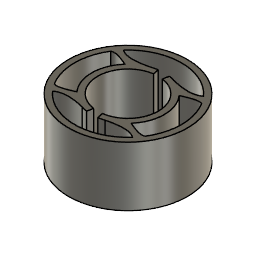
HeadTest (Autodesk Fusion 360 archive; units mm, degrees)
design "ReverseCoupler"
Autodesk Fusion 360 part; units mm, degrees
sketch "Sketch1" plane through (0, 0, 0) normal (0, 0, 1) x (1, 0, 0)
  circle A0 centre (0, 0) radius 5
  circle A1 centre (0, 0) radius 4.5
  line L0 (-6, 0) -> (8, 0) construction
  line L1 (0, -6.5) -> (0, 7.6827) construction
  line L2 (-0.3675, 2.5234) -> (-0.474, 3.0129)
  line L3 (-0.3675, -2.5234) -> (-0.474, -3.0129)
  line L4 (0.3675, -2.5234) -> (0.474, -3.0129)
  line L5 (0.3675, 2.5234) -> (0.474, 3.0129)
  arc A2 (-0.3675, 2.5234) -> (-0.3675, -2.5234) centre (0, 0) ccw
  arc A3 (0.3675, -2.5234) -> (0.3675, 2.5234) centre (0, 0) ccw
  arc A4 (-0.474, 3.0129) -> (-0.474, -3.0129) centre (0, 0) ccw
  arc A5 (0.474, -3.0129) -> (0.474, 3.0129) centre (0, 0) ccw
  spline S0 degree 5 poles (-0.9612, 2.8946) (-1.0282, 2.8783) (-1.1605, 2.8471) (-1.3543, 2.8051) (-1.6029, 2.7584) (-1.8962, 2.7168) (-2.1703, 2.6936) (-2.4235, 2.6906) (-2.6543, 2.7092) (-2.8628, 2.7492) (-3.0505, 2.8093) (-3.1851, 2.8722) (-3.2779, 2.9273) (-3.3362, 2.9674) (-3.3645, 2.9883) knots 0 0 0 0 0 0 0.1 0.2 0.3 0.4 0.5 0.6 0.7 0.8 0.9 1 1 1 1 1 1
  spline S1 degree 5 poles (-2.2886, 2.0162) (-2.3369, 2.0378) (-2.4322, 2.0797) (-2.5706, 2.1389) (-2.7462, 2.2105) (-2.9496, 2.2866) (-3.1354, 2.3481) (-3.3018, 2.3935) (-3.4472, 2.4215) (-3.5716, 2.4322) (-3.6763, 2.4265) (-3.7453, 2.4097) (-3.7893, 2.3907) (-3.8152, 2.3752) (-3.8273, 2.3668) knots 0 0 0 0 0 0 0.1 0.2 0.3 0.4 0.5 0.6 0.7 0.8 0.9 1 1 1 1 1 1
  spline S2 degree 5 poles (-0.9612, -2.8946) (-1.0282, -2.8783) (-1.1605, -2.8471) (-1.3543, -2.8051) (-1.6029, -2.7584) (-1.8962, -2.7168) (-2.1703, -2.6936) (-2.4235, -2.6906) (-2.6543, -2.7092) (-2.8628, -2.7492) (-3.0505, -2.8093) (-3.1851, -2.8722) (-3.2779, -2.9273) (-3.3362, -2.9674) (-3.3645, -2.9883) knots 0 0 0 0 0 0 0.1 0.2 0.3 0.4 0.5 0.6 0.7 0.8 0.9 1 1 1 1 1 1
  line L6 (-0.6756, 2.9642) -> (-1.2467, 2.825)
  line L7 (-3.1897, 2.8588) -> (-3.5393, 3.1178)
  line L8 (-0.6756, -2.9642) -> (-1.2467, -2.825)
  line L9 (-3.1897, -2.8588) -> (-3.5393, -3.1178)
  spline S3 degree 5 poles (-2.2886, -2.0162) (-2.3369, -2.0378) (-2.4322, -2.0797) (-2.5706, -2.1389) (-2.7462, -2.2105) (-2.9496, -2.2866) (-3.1354, -2.3481) (-3.3018, -2.3935) (-3.4472, -2.4215) (-3.5716, -2.4322) (-3.6763, -2.4265) (-3.7453, -2.4097) (-3.7893, -2.3907) (-3.8152, -2.3752) (-3.8273, -2.3668) knots 0 0 0 0 0 0 0.1 0.2 0.3 0.4 0.5 0.6 0.7 0.8 0.9 1 1 1 1 1 1
  line L10 (-2.0941, 1.9294) -> (-2.483, 2.1029)
  line L11 (-3.7334, 2.4323) -> (-3.9212, 2.3013)
  line L12 (-2.0941, -1.9294) -> (-2.483, -2.1029)
  line L13 (-3.7334, -2.4323) -> (-3.9212, -2.3013)
  spline S4 degree 5 poles (0.9612, 2.8946) (1.0282, 2.8783) (1.1605, 2.8471) (1.3543, 2.8051) (1.6029, 2.7584) (1.8962, 2.7168) (2.1703, 2.6936) (2.4235, 2.6906) (2.6543, 2.7092) (2.8628, 2.7492) (3.0505, 2.8093) (3.1851, 2.8722) (3.2779, 2.9273) (3.3362, 2.9674) (3.3645, 2.9883) knots 0 0 0 0 0 0 0.1 0.2 0.3 0.4 0.5 0.6 0.7 0.8 0.9 1 1 1 1 1 1
  line L14 (0.6756, 2.9642) -> (1.2467, 2.825)
  line L15 (3.1897, 2.8588) -> (3.5393, 3.1178)
  spline S5 degree 5 poles (2.2886, 2.0162) (2.3369, 2.0378) (2.4322, 2.0797) (2.5706, 2.1389) (2.7462, 2.2105) (2.9496, 2.2866) (3.1354, 2.3481) (3.3018, 2.3935) (3.4472, 2.4215) (3.5716, 2.4322) (3.6763, 2.4265) (3.7453, 2.4097) (3.7893, 2.3907) (3.8152, 2.3752) (3.8273, 2.3668) knots 0 0 0 0 0 0 0.1 0.2 0.3 0.4 0.5 0.6 0.7 0.8 0.9 1 1 1 1 1 1
  line L16 (2.0941, 1.9294) -> (2.483, 2.1029)
  line L17 (3.7334, 2.4323) -> (3.9212, 2.3013)
  spline S6 degree 5 poles (2.2886, -2.0162) (2.3369, -2.0378) (2.4322, -2.0797) (2.5706, -2.1389) (2.7462, -2.2105) (2.9496, -2.2866) (3.1354, -2.3481) (3.3018, -2.3935) (3.4472, -2.4215) (3.5716, -2.4322) (3.6763, -2.4265) (3.7453, -2.4097) (3.7893, -2.3907) (3.8152, -2.3752) (3.8273, -2.3668) knots 0 0 0 0 0 0 0.1 0.2 0.3 0.4 0.5 0.6 0.7 0.8 0.9 1 1 1 1 1 1
  line L18 (2.0941, -1.9294) -> (2.483, -2.1029)
  line L19 (3.7334, -2.4323) -> (3.9212, -2.3013)
  spline S7 degree 5 poles (0.9612, -2.8946) (1.0282, -2.8783) (1.1605, -2.8471) (1.3543, -2.8051) (1.6029, -2.7584) (1.8962, -2.7168) (2.1703, -2.6936) (2.4235, -2.6906) (2.6543, -2.7092) (2.8628, -2.7492) (3.0505, -2.8093) (3.1851, -2.8722) (3.2779, -2.9273) (3.3362, -2.9674) (3.3645, -2.9883) knots 0 0 0 0 0 0 0.1 0.2 0.3 0.4 0.5 0.6 0.7 0.8 0.9 1 1 1 1 1 1
  line L20 (0.6756, -2.9642) -> (1.2467, -2.825)
  line L21 (3.1897, -2.8588) -> (3.5393, -3.1178)
  point P0 (-2.5, 2.7)
  point P1 (-3.3645, 2.4039)
  point P2 (-2.5, -2.7)
  point P3 (-3.3645, -2.4039)
  point P4 (2.5, 2.7)
  point P5 (3.3645, 2.4039)
  point P6 (3.3645, -2.4039)
  point P7 (2.5, -2.7)
  dimension "d1" = 5.1
  dimension "d2" = 10
  dimension "d3" = -0.5
  constraint coincident A0.centre A1.centre
  constraint horizontal L0
  constraint vertical L1
  constraint symmetric L0 L2.start L3.start
  constraint symmetric L0 L2.end L3.end
  constraint symmetric L1 L2.start L5.start
  constraint symmetric L1 L2.end L5.end
  constraint symmetric L1 L3.start L4.start
  constraint symmetric L1 L3.end L4.end
  constraint concentric A2 A4
  constraint concentric A2 A3
  constraint concentric A4 A5
  constraint coincident A4 S0.start
  constraint coincident A1 S0.end
  constraint coincident A4 S1.start
  constraint coincident A1 S1.end
  constraint midpoint S0.start L6
  constraint midpoint S0.end L7
  constraint midpoint S1.start L10
  constraint midpoint S1.end L11
  constraint symmetric L0 S0.start S2.start
  constraint symmetric L0 P0 P2
  constraint symmetric L0 S0.end S2.end
  constraint symmetric L0 S1.start S3.start
  constraint symmetric L0 P1 P3
  constraint symmetric L0 S1.end S3.end
  constraint symmetric L0 L6.start L8.start
  constraint symmetric L0 L6.end L8.end
  constraint symmetric L0 L7.start L9.start
  constraint symmetric L0 L7.end L9.end
  constraint symmetric L0 L10.start L12.start
  constraint symmetric L0 L10.end L12.end
  constraint symmetric L0 L11.start L13.start
  constraint symmetric L0 L11.end L13.end
  constraint symmetric L1 S0.start S4.start
  constraint symmetric L1 P0 P4
  constraint symmetric L1 S0.end S4.end
  constraint symmetric L1 S1.start S5.start
  constraint symmetric L1 P1 P5
  constraint symmetric L1 S1.end S5.end
  constraint symmetric L1 S2.start S7.start
  constraint symmetric L1 P2 P7
  constraint symmetric L1 S2.end S7.end
  constraint symmetric L1 L6.start L14.start
  constraint symmetric L1 L6.end L14.end
  constraint symmetric L1 L7.start L15.start
  constraint symmetric L1 L7.end L15.end
  constraint symmetric L1 L8.start L20.start
  constraint symmetric L1 L8.end L20.end
  constraint symmetric L1 L9.start L21.start
  constraint symmetric L1 L9.end L21.end
  constraint symmetric L1 S3.start S6.start
  constraint symmetric L1 P3 P6
  constraint symmetric L1 S3.end S6.end
  constraint symmetric L1 L10.start L16.start
  constraint symmetric L1 L10.end L16.end
  constraint symmetric L1 L11.start L17.start
  constraint symmetric L1 L11.end L17.end
  constraint symmetric L1 L12.start L18.start
  constraint symmetric L1 L12.end L18.end
  constraint symmetric L1 L13.start L19.start
  constraint symmetric L1 L13.end L19.end
  measures "d1" diameter of A2
  measures "d2" diameter of A0
extrude "Extrude1" add sketch "Sketch1" along normal blind 3 contours A0 | A1 A5 S4 S5 L16 | A1 A5 S6 L18 S7 | A1 A4 S0 S1 L10 | L4 L5 A3 A5 | A1 A4 S2 S3 L12 | L2 L3 A2 A4
extrude "Extrude2" add 1 faces at (1.3362, -2.6414, 3) along direction (0, 0, 1) blind 5
extrude "Extrude3" cut 1 faces at (1.3362, -2.6414, 8) along direction (0, 0, -1) blind 3

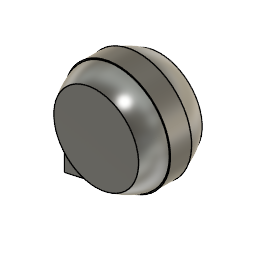
design "External1"
Autodesk Fusion 360 part; units mm, degrees
sketch "Sketch1" plane through (0, 0, 0) normal (0, 1, 0) x (1, 0, 0)
  circle A0 centre (5, -15) radius 10
  line L0 (-5, -15) -> (-5, -2.4877)
  line L1 (-5, -2.4877) -> (7.2045, -5.246)
  line L2 (5, -5) -> (5, -25)
  dimension "d1" = 20
  constraint coincident A0 L0.start
  constraint vertical L0
  constraint coincident A0 L1.end
  constraint tangent A0 L1
  constraint coincident A0 L2.start
  constraint coincident A0 L2.end
  constraint parallel L0 L2
  measures "d1" diameter of A0
revolve "Revolve1" add sketch "Sketch1" angle 360 about axis through (5, 0, 5) along (0, 0, 1) contours A0 L2 picked at (-0.5221, -14.2271)
extrude "Extrude1" add sketch "Sketch1" along normal mid plane 4
ref_plane "WorkPlane1" through (5, -1.184, 25) normal (0, 0, 1) x (-1, 0, 0)
sketch "Sketch2" plane through (0, 0, 25) normal (0, 0, 1) x (1, 0, 0)
  line L0 (-5, 10) -> (15, 10)
  line L1 (15, 10) -> (15, -10)
  line L2 (15, -10) -> (-5, -10)
  line L3 (-5, -10) -> (-5, 10)
  line L4 (-5, -6) -> (15, -6)
  line L5 (15, 6) -> (-5, 6)
  line L6 (-5, 0) -> (7.2045, 0)
  dimension "d8" = 6
  dimension "d9" = 6
  constraint horizontal L0
  constraint vertical L1
  constraint horizontal L2
  constraint vertical L3
  constraint coincident L3 L4.start
  constraint coincident L1 L4.end
  constraint perpendicular L1 L4
  constraint coincident L1 L5.start
  constraint coincident L3 L5.end
  constraint perpendicular L3 L5
  measures "d8" distance of L5 L6
  measures "d9" distance of L4 L6
extrude "Extrude2" cut sketch "Sketch2" against normal blind 27 contours L0 L1 L3 L5 | L1 L2 L3 L4
equation "d9 = d8"
